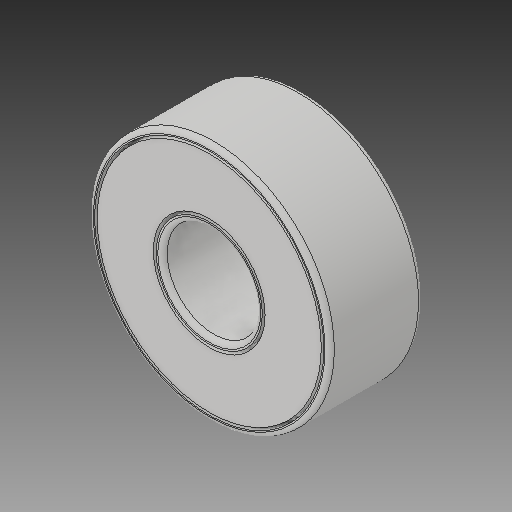
# Autodesk Inventor part: Ballbearing
Saved by Autodesk Inventor 2019 (Build 230136000, 136)
## iProperties
Created: 2024-10-15
Part Number: Ballbearing
Material: Generisch
Document SubType Name: Modeling
Designer: nic
Density: 1 g/cm^3
Appearance: Vorgabe
Author: nic
Autodesk Inventor part; units mm, degrees
ref_plane "YZ Plane" through (0, 0, 0) normal (1, 0, 0) x (0, 1, 0)
ref_plane "XZ Plane" through (0, 0, 0) normal (0, 1, 0) x (-1, 0, 0)
ref_plane "XY Plane" through (0, 0, 0) normal (0, 0, 1) x (1, 0, 0)
sketch "Skizze1" plane through (0, 0, 0) normal (0, 0, 1) x (1, 0, 0)
  circle A0 centre (0, 0) radius 2.575 construction
  circle A1 centre (0, 0) radius 1.45 construction
  circle A2 centre (0, 0) radius 2.575
  circle A3 centre (0, 0) radius 2.4485
  circle A4 centre (0, 0) radius 1
  circle A5 centre (0, 0) radius 1.1352
  point P0 (0, 0)
  dimension "d0" = 2
  constraints: 4 centre point, 2 coincident, 1 concentric
  measures "d0" diameter of A4
extrude "Extrusion1" add sketch "Skizze1" along normal blind 2
sketch "Skizze2" plane through (0, 0, 2) normal (0, 0, 1) x (1, 0, 0)
  circle A0 centre (0, 0) radius 1.1938
  circle A1 centre (0, 0) radius 2.3956
  constraints: 2 centre point, 1 coincident
extrude "Extrusion2" add sketch "Skizze2" against normal up to surface (2 mm away)
fillet "Rundung1" radius 0.1 2 edges at (-2.575, 0, 2) (-2.575, 0, 0)
fillet "Rundung2" radius 0.1 1 edges at (-1, 0, 2)
fillet "Rundung3" radius 0.1 1 edges at (-1, 0, 0)
